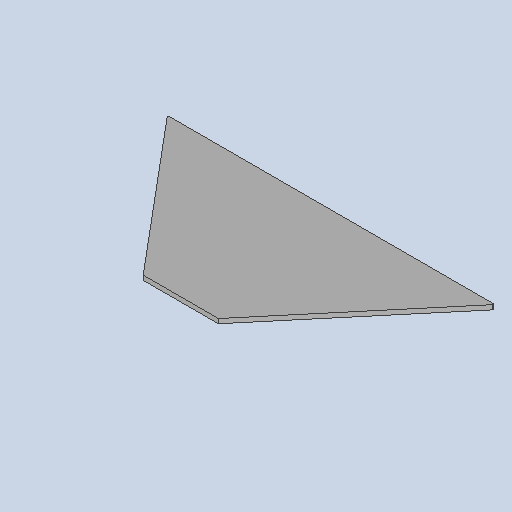
# Autodesk Inventor part: ДМФ 052 торец лотка кормовой
Saved by Autodesk Inventor 2025 (Build 290162010, 162A)
## iProperties
Created: 2024-05-13
Part Number: ДМФ 052 торец лотка кормовой
Material: Generic
Document SubType Name: Sheet Metal
Designer: admin
Density: 1 g/cm^3
Sheet Metal Rule: Default
Appearance: Default
Mass: 40.1707 g
Surface Area: 283.602 cm^2
Volume: 40.1707 cm^3
Flat Pattern Width: 10 cm
Flat Pattern Length: 21.6534 cm
Flat Pattern Area: 216.534 cm^2
Sheet Metal Width: 100,000 mm
Sheet Metal Length: 216,534 mm
Sheet Metal Area: 21653,435 mm^2
Author: admin
Autodesk Inventor part; units mm, degrees
ref_plane "YZ Plane" through (0, 0, 0) normal (1, 0, 0) x (0, 1, 0)
ref_plane "XZ Plane" through (0, 0, 0) normal (0, 1, 0) x (-1, 0, 0)
ref_plane "XY Plane" through (0, 0, 0) normal (0, 0, 1) x (1, 0, 0)
sketch "Sketch1" plane through (0, 0, 0) normal (0, 0, 1) x (1, 0, 0)
  line L0 (-108.91, 100) -> (-25, 0)
  line L1 (-25, 0) -> (25, 0)
  line L2 (25, 0) -> (108.91, 100)
  line L3 (108.91, 100) -> (-108.91, 100)
  point P0 (0, 0)
  point P1 (0, 0)
  point P2 (0, 100)
  dimension "BendRadius" = 3
  dimension "d0" = 100
  dimension "d1" = 50
  dimension "d2" = 217.8199
  dimension "d4" = 130
  measures "d0" distance between parallel lines of L1 L3
  measures "d1" distance of L0.end L1.end
  measures "d2" distance of L2.end L0.start
  measures "d4" angle of L1 L0
extrude "Plate1" add sketch "Sketch1" along normal blind 3
chamfer "Chamfer1" distance 1 angle 45 2 edges at (-108.91, 100, 1.5) (108.91, 100, 1.5)
equation "\"BendRadius\" = Thickness"
equation "\"d0\" = Лоток_высота"
equation "\"d1\" = Лоток_ширина_низ"
equation "\"d4\" = Лоток_угол"
equation "\"d3\" = Thickness"
equation "\"BendReliefWidth\" = Thickness"
equation "\"BendReliefDepth\" = 0.5 * Thickness"
equation "\"CornerReliefSize\" = 4 * Thickness"
equation "\"MinimumRemnant\" = 2 * Thickness"
equation "\"TransitionRadius\" = BendRadius"
equation "\"JacobiRadiusSize\" = BendRadius"
equation "\"GapSize\" = Thickness"
equation "\"Thickness\" = 3"
equation "\"Лоток_высота\" = 100"
equation "\"Лоток_ширина_низ\" = 50"
equation "\"Лоток_угол\" = 130deg"
body "Solid1"
